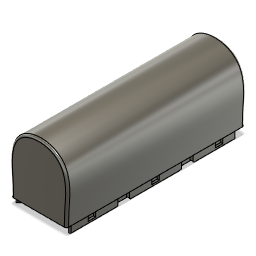
FimiPalm_18650 (Autodesk Fusion 360 design; units mm, degrees)
Autodesk Fusion 360 part; units mm, degrees
note: some values were not read from the file. Set by a fixed rule: which face or edge a step refers to.
sketch "Skizze1" plane through (0, 0, 0) normal (0, 0, 1) x (1, 0, 0)
  line L0 (0, 0) -> (0, 28) construction
  line L1 (0, 0) -> (11, 0) construction
  line L2 (0, 0) -> (-11, 0) construction
  line L3 (0, 16.5) -> (11.5, 16.5) construction
  line L4 (0, 16.5) -> (-11.5, 16.5) construction
  spline S0 degree 5 poles (-11, 0) (-11, 1.1184) (-11.0174, 3.2328) (-11.0955, 6.0367) (-11.2833, 9.0784) (-11.5268, 11.9443) (-11.6631, 14.2416) (-11.5466, 16.3578) (-11.2692, 18.8869) (-10.6013, 22.0051) (-8.7442, 25.1433) (-5.2316, 27.5376) (0, 28.4509) (5.2316, 27.5376) (8.7442, 25.1433) (10.6013, 22.0051) (11.2692, 18.8869) (11.5466, 16.3578) (11.6631, 14.2416) (11.5268, 11.9443) (11.2833, 9.0784) (11.0955, 6.0367) (11.0174, 3.2328) (11, 1.1184) (11, 0) knots 0 0 0 0 0 0 0.05 0.1 0.15 0.2 0.25 0.3 0.35 0.4 0.45 0.5 0.55 0.6 0.65 0.7 0.75 0.8 0.85 0.9 0.95 1 1 1 1 1 1
  line L5 (-11, -5) -> (-11, 5)
  line L6 (11, 5) -> (11, -5)
  line L7 (-4, 28) -> (4, 28)
  line L8 (-11.675, 14.5) -> (-11.325, 18.5)
  line L9 (11.325, 18.5) -> (11.675, 14.5)
  spline S1 degree 3 poles (-13, 0) (-13, 3.8211) (-13.1409, 6.7008) (-13.2975, 8.9494) (-13.4549, 11.2091) (-13.6198, 12.8876) (-13.6003, 14.571) (-13.5851, 15.8811) (-13.4917, 17.1438) (-13.2467, 18.7224) (-13.0529, 19.9702) (-12.7548, 21.4483) (-12.0503, 23.012) (-11.3266, 24.6184) (-10.1343, 26.2765) (-8.3658, 27.5415) (-6.5337, 28.852) (-4.0905, 29.7057) (-1.4947, 29.9345) (1.047, 30.1585) (3.693, 29.7959) (5.8931, 28.8969) (7.9509, 28.056) (9.5983, 26.7343) (10.722, 25.2564) (11.9595, 23.6287) (12.5818, 21.8567) (12.9353, 20.3456) (13.2936, 18.8138) (13.425, 17.5473) (13.5157, 16.3936) (13.6592, 14.5682) (13.5891, 12.9138) (13.436, 10.8422) (13.2918, 8.8912) (13.1034, 6.4965) (13.0325, 3.1971) (13.0113, 2.2103) (13, 1.1456) (13, 0) knots 0 0 0 0 0.103651 0.103651 0.103651 0.207815 0.207815 0.207815 0.288883 0.288883 0.288883 0.352962 0.352962 0.352962 0.418792 0.418792 0.418792 0.486989 0.486989 0.486989 0.553764 0.553764 0.553764 0.616219 0.616219 0.616219 0.684998 0.684998 0.684998 0.754718 0.754718 0.754718 0.86503 0.86503 0.86503 0.968924 0.968924 0.968924 1 1 1 1
  line L10 (-11, 0) -> (-13, 0)
  line L11 (11, 0) -> (13, 0)
  dimension "d5" = 23
  dimension "d6" = 22
  dimension "d7" = 5
  dimension "d8" = 8
  dimension "d9" = 4
  dimension "d10" = 10
  dimension "d11" = -2
  dimension "d12" = 11.5
  dimension "d13" = 28
  constraint coincident L0.start L1.start
  constraint vertical L0
  constraint perpendicular L0 L1
  constraint perpendicular L0 L2
  constraint equal L1 L2
  constraint coincident L0 L3.start
  constraint perpendicular L0 L3
  constraint perpendicular L0 L4
  constraint equal L3 L4
  constraint midpoint L2.end L5
  constraint vertical L5
  constraint midpoint L1.end L6
  constraint vertical L6
  constraint midpoint L0.end L7
  constraint horizontal L7
  constraint midpoint L4.end L8
  constraint midpoint L3.end L9
  constraint equal L8 L9
  constraint symmetric L0 L8 L9
  constraint parallel L2 L10
  constraint parallel L1 L11
  constraint equal L5 L6
  measures "d5" distance of L3.end L4.end
  measures "d6" distance of L1.end L2.end
  measures "d7" angle of L0 L8
  measures "d8" distance of L7.start L7.end
  measures "d9" vertical distance of L9.start L9.end
  measures "d10" distance of L6.start L6.end
  measures "d12" distance of L3 L7
  measures "d13" distance of L1 L7
extrude "Extrusion1" add sketch "Skizze1" along normal mid plane 84
extrude "Extrusion2" add 4 faces at (-11.6667, 0, 14) (-11.6667, 0, -14) (11.6667, 0, 14) (11.6667, 0, -14) along direction (0, -1, 0) blind 3
sketch "Skizze2" plane through (-13, 0, 0) normal (-1, 0, 0) x (0, 0, 1)
  line L0 (42, 0) -> (-42, 0)
  line L1 (-42, 0) -> (-42, -3)
  line L2 (-42, -3) -> (42, -3)
  line L3 (42, -3) -> (42, 0)
  line L4 (-1.75, -2.2) -> (1.75, -2.2)
  line L5 (1.75, -2.2) -> (1.75, 0)
  line L6 (1.75, 0) -> (-1.75, 0)
  line L7 (-1.75, 0) -> (-1.75, -2.2)
  line L8 (-1.75, -2.2) -> (1.75, 0) construction
  line L9 (1.75, -2.2) -> (-1.75, 0) construction
  point P0 (0, -1.1)
  dimension "d19" = 2.2
  dimension "d20" = 3.5
  constraint horizontal L4
  constraint perpendicular L4 L5
  constraint parallel L4 L6
  constraint parallel L5 L7
  constraint coincident L8 P0
  constraint coincident L9 P0
  constraint collinear L0 L6
  constraint vertical origin P0
  measures "d19" distance of L4.end L5.end
  measures "d20" distance of L4.start L4.end
extrude "Extrusion3" cut sketch "Skizze2" against normal blind 1 contours L0 L4 L5 L6 L7
pattern_linear "R-Anordnung1" count 3 spacing 30 along (0, 0, -1) both ways of "Extrusion3"
sketch "Skizze3" plane through (-13, 0, 0) normal (-1, 0, 0) x (0, 0, 1)
  line L0 (-31.75, -2.2) -> (-31.75, 0)
  line L1 (-31.75, 0) -> (-42, 0)
  line L2 (-42, 0) -> (-42, -3)
  line L3 (-42, -3) -> (42, -3)
  line L4 (42, -3) -> (42, 0)
  line L5 (42, 0) -> (31.75, 0)
  line L6 (31.75, 0) -> (31.75, -2.2)
  line L7 (31.75, -2.2) -> (28.25, -2.2)
  line L8 (28.25, -2.2) -> (28.25, 0)
  line L9 (28.25, 0) -> (1.75, 0)
  line L10 (1.75, 0) -> (1.75, -2.2)
  line L11 (1.75, -2.2) -> (-1.75, -2.2)
  line L12 (-1.75, -2.2) -> (-1.75, 0)
  line L13 (-1.75, 0) -> (-28.25, 0)
  line L14 (-28.25, 0) -> (-28.25, -2.2)
  line L15 (-28.25, -2.2) -> (-31.75, -2.2)
  line L16 (-28.25, -2.2) -> (-1.75, -2.2) construction
  line L17 (1.75, -2.2) -> (28.25, -2.2) construction
  line L18 (-15, -2.2) -> (-15, -1.5) construction
  line L19 (15, -2.2) -> (15, -1.5) construction
  line L20 (-12.25, -3) -> (-17.75, -3)
  line L21 (-17.75, -3) -> (-17.75, 0)
  line L22 (-17.75, 0) -> (-12.25, 0)
  line L23 (-12.25, 0) -> (-12.25, -3)
  line L24 (-12.25, -3) -> (-17.75, 0) construction
  line L25 (-17.75, -3) -> (-12.25, 0) construction
  line L26 (17.75, -3) -> (12.25, -3)
  line L27 (12.25, -3) -> (12.25, 0)
  line L28 (12.25, 0) -> (17.75, 0)
  line L29 (17.75, 0) -> (17.75, -3)
  line L30 (17.75, -3) -> (12.25, 0) construction
  line L31 (12.25, -3) -> (17.75, 0) construction
  point P0 (-15, -1.5)
  point P1 (15, -1.5)
  dimension "d29" = 5.5
  constraint coincident L14.end L15.start
  constraint coincident L11.end L12.start
  constraint coincident L10.end L11.start
  constraint coincident L7.end L8.start
  constraint midpoint L16 L18.start
  constraint perpendicular L16 L18
  constraint midpoint L17 L19.start
  constraint perpendicular L17 L19
  constraint horizontal L20
  constraint perpendicular L20 L21
  constraint parallel L20 L22
  constraint parallel L21 L23
  constraint coincident L3 L20.start
  constraint coincident L24 P0
  constraint coincident L25 P0
  constraint coincident P0 L18.end
  constraint horizontal L26
  constraint perpendicular L26 L27
  constraint parallel L26 L28
  constraint parallel L27 L29
  constraint coincident L3 L26.start
  constraint coincident L30 P1
  constraint coincident L31 P1
  constraint coincident P1 L19.end
  constraint collinear L9 L28
  constraint collinear L13 L22
  constraint equal L22 L28
  measures "d29" distance of L21.end L22.end
extrude "Extrusion4" cut sketch "Skizze3" against normal blind 1.5 contours L3 L13 L20 L21 L22 L23 | L3 L9 L26 L27 L28 L29
fillet "Abrundung1" radius 0.5 4 edges at (-12.25, -3, -17.75) (-12.25, -3, -12.25) (-12.25, -3, 12.25) (-12.25, -3, 17.75)
mirror "Spiegeln2" about plane through (0, 0, 0) normal (1, 0, 0) of "Extrusion3", "R-Anordnung1", "Extrusion4", "Abrundung1"
sketch "Skizze4" plane through (0, 0, 42) normal (0, 0, 1) x (1, 0, 0)
  spline S0 degree 5 poles (-11, 0) (-11, 1.1184) (-11.0174, 3.2328) (-11.0955, 6.0367) (-11.2833, 9.0784) (-11.5268, 11.9443) (-11.6631, 14.2416) (-11.5466, 16.3578) (-11.2692, 18.8869) (-10.6013, 22.0051) (-8.7442, 25.1433) (-5.2316, 27.5376) (0, 28.4509) (5.2316, 27.5376) (8.7442, 25.1433) (10.6013, 22.0051) (11.2692, 18.8869) (11.5466, 16.3578) (11.6631, 14.2416) (11.5268, 11.9443) (11.2833, 9.0784) (11.0955, 6.0367) (11.0174, 3.2328) (11, 1.1184) (11, 0) knots 0 0 0 0 0 0 0.05 0.1 0.15 0.2 0.25 0.3 0.35 0.4 0.45 0.5 0.55 0.6 0.65 0.7 0.75 0.8 0.85 0.9 0.95 1 1 1 1 1 1
  line L0 (11, 0) -> (11, -3)
  line L1 (11, -3) -> (13, -3)
  line L2 (13, -3) -> (13, 0)
  spline S1 degree 3 poles (13, 0) (13, 1.1456) (13.0113, 2.2103) (13.0325, 3.1971) (13.1034, 6.4965) (13.2918, 8.8912) (13.436, 10.8422) (13.5891, 12.9138) (13.6592, 14.5682) (13.5157, 16.3936) (13.425, 17.5473) (13.2936, 18.8138) (12.9353, 20.3456) (12.5818, 21.8567) (11.9595, 23.6287) (10.722, 25.2564) (9.5983, 26.7343) (7.9509, 28.056) (5.8931, 28.8969) (3.693, 29.7959) (1.047, 30.1585) (-1.4947, 29.9345) (-4.0905, 29.7057) (-6.5337, 28.852) (-8.3658, 27.5415) (-10.1343, 26.2765) (-11.3266, 24.6184) (-12.0503, 23.012) (-12.7548, 21.4483) (-13.0529, 19.9702) (-13.2467, 18.7224) (-13.4917, 17.1438) (-13.5851, 15.8811) (-13.6003, 14.571) (-13.6198, 12.8876) (-13.4549, 11.2091) (-13.2975, 8.9494) (-13.1409, 6.7008) (-13, 3.8211) (-13, 0) knots -1 -1 -1 -1 -0.968924 -0.968924 -0.968924 -0.86503 -0.86503 -0.86503 -0.754718 -0.754718 -0.754718 -0.684998 -0.684998 -0.684998 -0.616219 -0.616219 -0.616219 -0.553764 -0.553764 -0.553764 -0.486989 -0.486989 -0.486989 -0.418792 -0.418792 -0.418792 -0.352962 -0.352962 -0.352962 -0.288883 -0.288883 -0.288883 -0.207815 -0.207815 -0.207815 -0.103651 -0.103651 -0.103651 0 0 0 0
  line L3 (-13, 0) -> (-13, -3)
  line L4 (-13, -3) -> (-11, -3)
  line L5 (-11, -3) -> (-11, 0)
  line L6 (-11, -3) -> (11, -3)
  constraint coincident L4.end L5.start
  constraint coincident L0.end L1.start
extrude "Extrusion5" add sketch "Skizze4" against normal blind 1 contours S0 L0 L5 L6
fillet "Abrundung2" radius 2 3 edges at (11, -1.5, 41) (1.3678, 27.9379, 41) (-11, -1.5, 41)
fillet "Abrundung3" radius 1 3 edges at (13, -1.5, 42) (-0.0011, 29.999, 42) (-13, -1.5, 42)
sketch "Skizze5" plane through (0, 0, -42) normal (0, 0, -1) x (-1, 0, 0)
  spline S0 degree 5 poles (-11, 0) (-11, 1.1184) (-11.0174, 3.2328) (-11.0955, 6.0367) (-11.2833, 9.0784) (-11.5268, 11.9443) (-11.6631, 14.2416) (-11.5466, 16.3578) (-11.2692, 18.8869) (-10.6013, 22.0051) (-8.7442, 25.1433) (-5.2316, 27.5376) (0, 28.4509) (5.2316, 27.5376) (8.7442, 25.1433) (10.6013, 22.0051) (11.2692, 18.8869) (11.5466, 16.3578) (11.6631, 14.2416) (11.5268, 11.9443) (11.2833, 9.0784) (11.0955, 6.0367) (11.0174, 3.2328) (11, 1.1184) (11, 0) knots -1 -1 -1 -1 -1 -1 -0.95 -0.9 -0.85 -0.8 -0.75 -0.7 -0.65 -0.6 -0.55 -0.5 -0.45 -0.4 -0.35 -0.3 -0.25 -0.2 -0.15 -0.1 -0.05 0 0 0 0 0 0
  line L0 (11, 0) -> (11, -3)
  line L1 (11, -3) -> (13, -3)
  line L2 (13, -3) -> (13, 0)
  spline S1 degree 3 poles (13, 0) (13, 3.8211) (13.1409, 6.7008) (13.2975, 8.9494) (13.4549, 11.2091) (13.6198, 12.8876) (13.6003, 14.571) (13.5851, 15.8811) (13.4917, 17.1438) (13.2467, 18.7224) (13.0529, 19.9702) (12.7548, 21.4483) (12.0503, 23.012) (11.3266, 24.6184) (10.1343, 26.2765) (8.3658, 27.5415) (6.5337, 28.852) (4.0905, 29.7057) (1.4947, 29.9345) (-1.047, 30.1585) (-3.693, 29.7959) (-5.8931, 28.8969) (-7.9509, 28.056) (-9.5983, 26.7343) (-10.722, 25.2564) (-11.9595, 23.6287) (-12.5818, 21.8567) (-12.9353, 20.3456) (-13.2936, 18.8138) (-13.425, 17.5473) (-13.5157, 16.3936) (-13.6592, 14.5682) (-13.5891, 12.9138) (-13.436, 10.8422) (-13.2918, 8.8912) (-13.1034, 6.4965) (-13.0325, 3.1971) (-13.0113, 2.2103) (-13, 1.1456) (-13, 0) knots 0 0 0 0 0.103651 0.103651 0.103651 0.207815 0.207815 0.207815 0.288883 0.288883 0.288883 0.352962 0.352962 0.352962 0.418792 0.418792 0.418792 0.486989 0.486989 0.486989 0.553764 0.553764 0.553764 0.616219 0.616219 0.616219 0.684998 0.684998 0.684998 0.754718 0.754718 0.754718 0.86503 0.86503 0.86503 0.968924 0.968924 0.968924 1 1 1 1
  line L3 (-13, 0) -> (-13, -3)
  line L4 (-13, -3) -> (-11, -3)
  line L5 (-11, -3) -> (-11, 0)
  line L6 (-11, -3) -> (11, -3)
  constraint coincident L4.end L5.start
  constraint coincident L0.end L1.start
extrude "Extrusion6" add sketch "Skizze5" against normal blind 1 contours S0 L0 L5 L6
fillet "Abrundung4" radius 7 3 edges at (-11, -1.5, -41) (-1.3678, 27.9379, -41) (11, -1.5, -41)
fillet "Abrundung5" radius 1 3 edges at (-13, -1.5, -42) (-0.0011, 29.999, -42) (13, -1.5, -42)
sketch "Skizze6" plane through (0, -3, 0) normal (0, -1, 0) x (1, 0, 0)
  arc A0 (-13, -41) -> (-12, -42) centre (-12, -41) ccw
  line L0 (-12, -42) -> (12, -42)
  arc A1 (12, -42) -> (13, -41) centre (12, -41) ccw
  line L1 (13, -41) -> (13, -18.25)
  line L2 (13, -18.25) -> (11.5, -18.25)
  line L3 (11, 39) -> (11, -34)
  arc A2 (4, -41) -> (11, -34) centre (4, -34) ccw
  line L4 (4, -41) -> (-4, -41)
  arc A3 (-11, -34) -> (-4, -41) centre (-4, -34) ccw
  line L5 (-11, -34) -> (-11, 39)
  line L6 (-11.5, -18.25) -> (-13, -18.25)
  line L7 (-13, 41) -> (-13, 18.25)
  line L8 (12, 42) -> (-12, 42)
  arc A4 (-12, 42) -> (-13, 41) centre (-12, 41) ccw
  line L9 (-13, 41) -> (-13, 18.25)
  line L10 (-13, 18.25) -> (-11.5, 18.25)
  line L11 (-11, -34) -> (-11, 39)
  arc A5 (-9, 41) -> (-11, 39) centre (-9, 39) ccw
  line L12 (-9, 41) -> (9, 41)
  arc A6 (11, 39) -> (9, 41) centre (9, 39) ccw
  line L13 (11, 39) -> (11, -34)
  line L14 (11.5, 18.25) -> (13, 18.25)
  line L15 (13, -41) -> (13, -18.25)
  line L16 (11, -34) -> (13, -41)
  line L17 (11.5, -18.25) -> (11.5, -11.75)
  line L18 (11.5, -11.75) -> (13, -11.75)
  line L19 (13, -11.75) -> (13, 11.75)
  line L20 (13, 11.75) -> (11.5, 11.75)
  line L21 (11.5, 11.75) -> (11.5, 18.25)
  line L22 (11.5, 18.25) -> (13, 18.25)
  line L23 (13, 18.25) -> (13, 41)
  line L24 (12, 42) -> (-12, 42)
  arc A7 (-12, 42) -> (-13, 41) centre (-12, 41) ccw
  line L25 (-13, 18.25) -> (-11.5, 18.25)
  line L26 (-11.5, 18.25) -> (-11.5, 11.75)
  line L27 (-11.5, 11.75) -> (-13, 11.75)
  line L28 (-13, 11.75) -> (-13, -11.75)
  line L29 (-13, -11.75) -> (-11.5, -11.75)
  line L30 (-11.5, -11.75) -> (-11.5, -18.25)
  arc A8 (-9, 41) -> (-11, 39) centre (-9, 39) ccw
  line L31 (-9, 41) -> (9, 41)
  arc A9 (11, 39) -> (9, 41) centre (9, 39) ccw
  arc A10 (12, -42) -> (13, -41) centre (12, -41) ccw
  line L32 (13, -18.25) -> (11.5, -18.25)
  line L33 (11.5, -18.25) -> (11.5, -11.75)
  line L34 (11.5, -11.75) -> (13, -11.75)
  line L35 (13, -11.75) -> (13, 11.75)
  line L36 (13, 11.75) -> (11.5, 11.75)
  line L37 (11.5, 11.75) -> (11.5, 18.25)
  line L38 (-11.5, 18.25) -> (-11.5, 11.75)
  line L39 (-11.5, 11.75) -> (-13, 11.75)
  line L40 (-13, 11.75) -> (-13, -11.75)
  line L41 (-13, -11.75) -> (-11.5, -11.75)
  line L42 (-11.5, -11.75) -> (-11.5, -18.25)
  line L43 (-11.5, -18.25) -> (-13, -18.25)
  line L44 (-13, -18.25) -> (-13, -41)
  arc A11 (-13, -41) -> (-12, -42) centre (-12, -41) ccw
  line L45 (-12, -42) -> (12, -42)
  arc A12 (4, -41) -> (11, -34) centre (4, -34) ccw
  line L46 (4, -41) -> (-4, -41)
  arc A13 (-11, -34) -> (-4, -41) centre (-4, -34) ccw
  line L47 (-11, 39) -> (-13, 41)
  line L48 (11, 39) -> (13, 41)
  line L49 (-11, -34) -> (-13, -41)
  arc A14 (-12, 42) -> (-13, 41) centre (-12, 41) ccw
  line L50 (-12.602, 42) -> (12.5939, 42)
  arc A15 (13, 41) -> (12, 42) centre (12, 41) ccw
  line L51 (13.5939, 41) -> (-13.6021, 41)
  line L52 (-13, -18.25) -> (-13, -41)
  line L53 (13, 18.25) -> (13, 41)
  constraint coincident L3.end A2.end
  constraint coincident A1.end L1.start
  constraint coincident L5.end L11.end
  constraint coincident L7.start A4.end
  constraint coincident L3.start A6.start
  constraint coincident A3.start L5.start
  constraint coincident A0.start L44.end
  constraint coincident L23.end L48.end
extrude "Extrusion7" cut sketch "Skizze6" against normal blind 3 contours A0 L0 A1 A2 L4 A3 L16 A10 A11 L45 A12 L46 A13 L49 | A5 A8 L47 L51 | L8 A4 L12 L24 A7 L31 A14 L50 A15 L51 | A6 A9 L48 L51
fillet "Abrundung6" radius 0.5 4 edges at (13, -1.5, -41) (-13, -1.5, -41) (13, -1.5, 41) (-13, -1.5, 41)
sketch "Skizze7" plane through (0, 0, 0) normal (0, -1, 0) x (1, 0, 0)
  line L0 (4, -41) -> (-4, -41)
  arc A0 (-11, -34) -> (-4, -41) centre (-4, -34) ccw
  line L1 (-13, -37.43) -> (-13, -41)
  arc A1 (-13, -41) -> (-12, -42) centre (-12, -41) ccw
  line L2 (-12, -42) -> (12, -42)
  arc A2 (4, -41) -> (11, -34) centre (4, -34) ccw
  line L3 (4.5, -42) -> (-4.5, -42)
  line L4 (-4.5, -42) -> (-4.5, -40.5)
  line L5 (-4.5, -40.5) -> (4.5, -40.5)
  line L6 (4.5, -40.5) -> (4.5, -42)
  line L7 (4.5, -42) -> (-4.5, -40.5) construction
  line L8 (-4.5, -42) -> (4.5, -40.5) construction
  line L9 (-11, -34) -> (-12.0192, -37.5673)
  arc A3 (-13, -37.43) -> (-12.0192, -37.5673) centre (-12.5, -37.43) ccw
  arc A4 (12, -42) -> (13, -41) centre (12, -41) ccw
  line L10 (13, -41) -> (13, -37.43)
  arc A5 (12.0192, -37.5673) -> (13, -37.43) centre (12.5, -37.43) ccw
  line L11 (12.0192, -37.5673) -> (11, -34)
  point P0 (0, -41.25)
  dimension "d53" = 9
  dimension "d56" = 1.5
  constraint horizontal L3
  constraint perpendicular L3 L4
  constraint parallel L3 L5
  constraint parallel L4 L6
  constraint coincident L7 P0
  constraint coincident L8 P0
  constraint vertical origin P0
  constraint collinear L2 L3
  measures "d53" distance of L4.end L5.end
  measures "d56" distance of L3 L5
extrude "Extrusion8" cut sketch "Skizze7" against normal blind 2 contours L0 A0 L2 A2 L3 L4 L6 | L0 A0 A2 L4 L5 L6
fillet "Abrundung7" radius 1 4 edges at (-4.5, 0, -41.4911) (4.5, 0, -41.4911) (-4.5, 2, -41.4915) (4.5, 2, -41.4915)
equation "d12 = d5 / 2"
